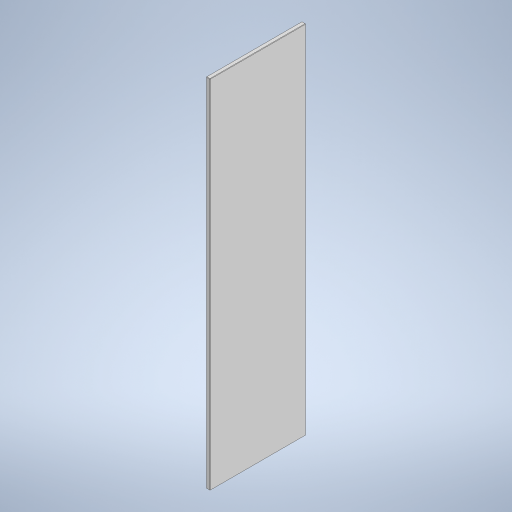
# Autodesk Inventor part: floor
Saved by Autodesk Inventor 2024 (Build 280153000, 153)
## iProperties
Created: 2025-11-21
Part Number: floor
Material: Generic
Document SubType Name: Modeling
Designer: dearl
Density: 1 g/cm^3
Appearance: Default
Author: dearl
Autodesk Inventor part; units mm, degrees
ref_plane "YZ Plane" through (0, 0, 0) normal (1, 0, 0) x (0, 1, 0)
ref_plane "XZ Plane" through (0, 0, 0) normal (0, 1, 0) x (-1, 0, 0)
ref_plane "XY Plane" through (0, 0, 0) normal (0, 0, 1) x (1, 0, 0)
sketch "Sketch1" plane through (0, 0, 0) normal (0, 1, 0) x (-1, 0, 0)
  line L0 (0, 0) -> (1, 0)
  line L1 (1, 0) -> (1, -24.5)
  line L2 (1, -24.5) -> (0, -24.5)
  line L3 (0, -24.5) -> (0, 0)
  dimension "d0" = 1
  dimension "d1" = 24.5
  constraints: 8 end point, 2 parallel, 1 horizontal, 1 perpendicular
  measures "d0" distance of L1.end L2.end
  measures "d1" distance of L0.end L1.end
extrude "Extrusion1" add sketch "Sketch1" along normal blind 91.1
chamfer "Chamfer1" distance 0.1 angle 45 8 edges at (0, 91.1, -12.25) (-1, 91.1, -12.25) (0, 0, -12.25) (-1, 0, -12.25) (-0.5, 91.1, 0) (-0.5, 91.1, -24.5) (-0.5, 0, 0) (-0.5, 0, -24.5)
fillet "Fillet1" radius 0.1 4 edges at (-1, 45.55, 0) (0, 45.55, 0) (-1, 45.55, -24.5) (0, 45.55, -24.5)
body "Solid1"
